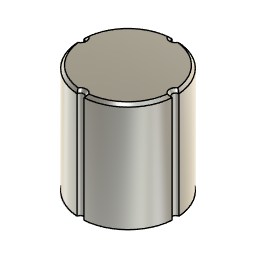
Assembly (Autodesk Fusion 360 archive; units mm, degrees)
design "Part2"
Autodesk Fusion 360 part; units mm, degrees
sketch "Sketch1" plane through (0, 0, 0) normal (0, 0, 1) x (1, 0, 0)
  circle A0 centre (0, 0) radius 3.5
  circle A1 centre (0, 0) radius 2.5
  line L0 (-2, 1.5) -> (2, 1.5)
  line L1 (-2, -1.5) -> (2, -1.5)
  circle A2 centre (3.5, 0) radius 0.25
  circle A3 centre (0, 3.5) radius 0.25
  circle A4 centre (-3.5, 0) radius 0.25
  circle A5 centre (0, -3.5) radius 0.25
  dimension "d1" = 7
  dimension "d2" = 5
  dimension "d3" = 3
  dimension "d4" = 1.5
  dimension "d12" = 0.5
  dimension "d13" = 0.5
  dimension "d14" = 0.5
  dimension "d15" = 0.5
  constraint coincident A0.centre A1.centre
  constraint concentric A0 A1
  constraint coincident A1 L0.start
  constraint coincident A1 L0.end
  constraint horizontal L0
  constraint coincident A1 L1.start
  constraint coincident A1 L1.end
  constraint parallel L0 L1
  constraint coincident A0 A2.centre
  constraint coincident A0 A3.centre
  constraint coincident A0 A4.centre
  constraint coincident A0 A5.centre
  measures "d1" diameter of A0
  measures "d2" diameter of A1
  measures "d3" distance of L0 L1
  measures "d4" distance of A0.centre L1
  measures "d12" diameter of A2
  measures "d13" diameter of A3
  measures "d14" diameter of A4
  measures "d15" diameter of A5
extrude "Extrude1" add sketch "Sketch1" along normal blind 8 contours A0 A2 A3 A4 A5 | A1 L0 L1 | A1 L0 | A1 L1
extrude "Extrude2" cut sketch "Sketch1" along normal blind 1 contours A1 L0 L1 | A1 L0 | A1 L1
extrude "Extrude3" cut sketch "Sketch1" along normal blind 7 contours A1 L0 L1
chamfer "Chamfer2" distance 0.2 angle 45 8 edges at (-2.4749, 2.4749, 8) (-3.25, 0, 8) (-2.4749, -2.4749, 8) (0, -3.25, 8) (2.4749, -2.4749, 8) (3.25, 0, 8) (2.4749, 2.4749, 8) (0, 3.25, 8)
